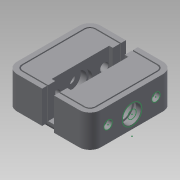
# Autodesk Inventor part: Sepatu
Saved by Autodesk Inventor 2015 SP1 (Build 190203100, 203)
## iProperties
Created: 2015-02-21
Part Number: Sepatu
Material: Generic
Document SubType Name: Modeling
Designer: Rafi Kurnia Putra
Density: 1 g/cm^3
Appearance: Default
Author: Rafi Kurnia Putra
Autodesk Inventor part; units mm, degrees
note: some values were not read from the file. Chosen so that the rebuilt part matches the saved one: copy form of "Mirror3".
ref_plane "YZ Plane" through (0, 0, 0) normal (1, 0, 0) x (0, 1, 0)
ref_plane "XZ Plane" through (0, 0, 0) normal (0, 1, 0) x (-1, 0, 0)
sketch "Sketch1" plane through (0, 0, 0) normal (0, 1, 0) x (-1, 0, 0)
  line L0 (-15, 15) -> (15, 15)
  line L1 (15, -15) -> (-15, -15)
  line L2 (-15, 15) -> (15, -15) construction
  line L3 (15, 15) -> (-15, -15) construction
  line L4 (15, 15) -> (15, 2.5)
  line L5 (15, -2.5) -> (15, -15)
  line L6 (-15, -15) -> (-15, -2.5)
  line L7 (-15, 2.5) -> (-15, 15)
  line L8 (12, 2.5) -> (12, 12)
  line L9 (12, 12) -> (-12, 12)
  line L10 (-12, 12) -> (-12, 2.5)
  line L11 (12, -2.5) -> (12, -12)
  line L12 (12, -12) -> (-12, -12)
  line L13 (-12, -12) -> (-12, -2.5)
  line L14 (15, 2.5) -> (12, 2.5)
  line L15 (15, -2.5) -> (12, -2.5)
  line L16 (-12, 2.5) -> (-15, 2.5)
  line L17 (-12, -2.5) -> (-15, -2.5)
  line L18 (12, 2.5) -> (12, -2.5)
  line L19 (-12, 2.5) -> (-12, -2.5)
  line L20 (15, -2.5) -> (15, 2.5)
  line L21 (-15, -2.5) -> (-15, 2.5)
  point P0 (0, 0)
  point P1 (15, -2.5)
  dimension "d0" = 30
  dimension "d1" = 30
  constraints: 44 end point, 9 parallel, 5 horizontal, 3 perpendicular, 2 midpoint, 2 vertical, 4 other
  measures "d0" distance of L1.start L1.end
  measures "d1" distance of L0.end L1.start
extrude "Extrusion1" add sketch "Sketch1" along normal blind 3 contours L10 L9 L8 L18 L11 L12 L13 L19
extrude "Extrusion2" add sketch "Sketch1" along normal blind 30 contours L0 L4 L14 L8 L9 L10 L16 L7 | L17 L13 L12 L11 L15 L5 L1 L6
extrude "Extrusion3" add sketch "Sketch1" along normal blind 3 contours L16 L19 L17 L21 | L20 L15 L18 L14
sketch "Sketch2" plane through (-15, 0, 15) normal (0, 0, 1) x (1, 0, 0)
  circle A0 centre (15, 8) radius 5
  line L0 (0, 0) -> (30, 0) projected
  circle A1 centre (15, 8) radius 1.75
  circle A2 centre (15, 8) radius 4.125
  dimension "d8" = 10
  dimension "d9" = 8
  dimension "d12" = 3.5
  dimension "d21" = 8.25
  constraints: 3 centre point, 2 coincident
  measures "d8" diameter of A0
  measures "d9" distance from line of L0 A0.centre
  measures "d12" diameter of A1
  measures "d21" diameter of A2
extrude "Extrusion6" add sketch "Sketch2" against normal blind 11 contours A0 | A1 | A2
extrude "Extrusion7" cut sketch "Sketch2" against normal up to next contours A1
extrude "Extrusion8" cut sketch "Sketch2" against normal blind 1.5 contours A0 | A2
extrude "Extrusion9" cut sketch "Sketch2" against normal blind 4 contours A1 | A2
fillet "Fillet1" radius 2 4 edges at (15, 0, 0) (0, 0, 15) (0, 0, -15) (-15, 0, 0)
fillet "Fillet2" radius 2 8 edges at (14.4142, 0.5858, 14.4142) (15, 16, 15) (14.4142, 0.5858, -14.4142) (15, 16, -15) (-14.4142, 0.5858, -14.4142) (-15, 16, -15) (-14.4142, 0.5858, 14.4142) (-15, 16, 15)
ref_plane "Work Plane1" through (0, 0, 9.5) normal (0, 0, 1) x (1, 0, 0)
mirror "Mirror3" about plane through (0, 0, 9.5) normal (0, 0, 1) of "Extrusion8", "Extrusion9", "Extrusion7" geometry pattern yes
mirror "Mirror4" about plane through (0, 0, 0) normal (0, 0, 1) of "Extrusion8", "Extrusion9", "Extrusion6", "Extrusion7", "Mirror3"
sketch "Sketch6" plane through (0, 30, 0) normal (0, 1, 0) x (1, 0, 0)
  line L0 (-15, -2.5) -> (-15, -13) projected
  arc A0 (-15, -13) -> (-13, -15) centre (-13, -13) ccw projected
  line L1 (-13, -15) -> (13, -15) projected
  arc A1 (13, -15) -> (15, -13) centre (13, -13) ccw projected
  line L2 (15, -13) -> (15, -2.5) projected
  line L3 (15, 2.5) -> (15, 13) projected
  arc A2 (15, 13) -> (13, 15) centre (13, 13) ccw projected
  line L4 (13, 15) -> (-13, 15) projected
  arc A3 (-13, 15) -> (-15, 13) centre (-13, 13) ccw projected
  line L5 (-15, 13) -> (-15, 2.5) projected
  line L6 (15.5, -2.5) -> (15.5, -13)
  arc A4 (13, -15.5) -> (15.5, -13) centre (13, -13) ccw
  line L7 (13, -15.5) -> (-13, -15.5)
  arc A5 (-15.5, -13) -> (-13, -15.5) centre (-13, -13) ccw
  line L8 (-15.5, -13) -> (-15.5, -2.5)
  line L9 (-15.5, 2.5) -> (-15.5, 13)
  arc A6 (-13, 15.5) -> (-15.5, 13) centre (-13, 13) ccw
  line L10 (-13, 15.5) -> (13, 15.5)
  arc A7 (15.5, 13) -> (13, 15.5) centre (13, 13) ccw
  line L11 (15.5, 13) -> (15.5, 2.5)
  line L12 (-17.5, -2.5) -> (-17.5, -13)
  arc A8 (-17.5, -13) -> (-13, -17.5) centre (-13, -13) ccw
  line L13 (-13, -17.5) -> (13, -17.5)
  arc A9 (13, -17.5) -> (17.5, -13) centre (13, -13) ccw
  line L14 (17.5, -13) -> (17.5, -2.5)
  line L15 (17.5, 2.5) -> (17.5, 13)
  arc A10 (17.5, 13) -> (13, 17.5) centre (13, 13) ccw
  line L16 (13, 17.5) -> (-13, 17.5)
  arc A11 (-13, 17.5) -> (-17.5, 13) centre (-13, 13) ccw
  line L17 (-17.5, 13) -> (-17.5, 2.5)
  line L18 (17.5, -2.5) -> (15.5, -2.5)
  line L19 (-15.5, -2.5) -> (-17.5, -2.5)
  line L20 (-15.5, 2.5) -> (-17.5, 2.5)
  line L21 (17.5, 2.5) -> (15.5, 2.5)
  point P0 (0, 0)
  dimension "d38" = 0.5
  dimension "d39" = 0.5
  dimension "d40" = 2
  dimension "d41" = 2
  constraints: 32 end point, 16 point on circle, 8 centre point, 2 horizontal, 1 parallel, 1 perpendicular, 16 other
  measures "d38" distance between parallel lines of L6 L2
  measures "d39" distance between parallel lines of L3 L11
  measures "d40" distance between parallel lines of L7 L13
  measures "d41" distance between parallel lines of L10 L16
extrude "Extrusion11" add sketch "Sketch6" against normal blind 27.5
sketch "Sketch10" plane through (-13, 30, 17.5) normal (0, 0, 1) x (1, 0, 0)
  line L0 (26, -27.5) -> (0, -27.5) projected
  circle A0 centre (13, -22) radius 1.75 projected
  line L1 (0, -30) -> (26, -30) projected
  line L2 (30.5, 0) -> (30.5, -27.5) projected
  line L3 (-4.5, 0) -> (30.5, 0)
  line L4 (30.5, 0) -> (30.5, -14)
  line L5 (30.5, -14) -> (-4.5, -14)
  line L6 (-4.5, -14) -> (-4.5, 0)
  point P0 (13, -30)
  point P1 (13, -14)
  dimension "d51" = 5.5
  dimension "d52" = 8
  constraints: 8 end point, 2 parallel, 1 horizontal, 1 perpendicular, 1 point on line
  measures "d51" distance from line of L0 A0.centre
  measures "d52" distance of point (13, -14) A0.centre
extrude "Extrusion15" cut sketch "Sketch10" against normal through all contours L2 L5 L6 L3
sketch "Sketch11" plane through (-13, 2.5, 17.5) normal (0, 0, 1) x (1, 0, 0)
  circle A0 centre (13, 5.5) radius 4.125 projected
  circle A1 centre (13, 5.5) radius 3.75
  point P0 (13, -2.5)
  dimension "d55" = 7.5
  constraints: 1 centre point, 1 coincident
  measures "d55" diameter of A1
extrude "Extrusion16" cut sketch "Sketch11" against normal blind 2 contours A1
mirror "Mirror7" about plane through (0, 0, 0) normal (0, 0, 1) of "Extrusion16"
sketch "Sketch12" plane through (13, 2.5, -17.5) normal (0, 0, -1) x (-1, 0, 0)
  circle A0 centre (13, 5.5) radius 3.75 projected
  line L0 (26, 13.5) -> (0, 13.5) projected
  line L1 (0, 13.5) -> (0, 0) projected
  line L2 (26, 0) -> (0, 0) projected
  line L3 (26, 13.5) -> (26, 0) projected
  line L4 (0, 13.5) -> (26, 0) construction
  line L5 (26, 0) -> (26, 13.5)
  line L6 (26, 13.5) -> (26, 0) projected
  line L7 (26, 13.5) -> (0, 0) construction
  line L8 (0, 0) -> (13, 6.75) construction
  line L9 (13, 12.25) -> (13, 6.75) construction
  line L10 (-2, 0.5) -> (1, 0.5) projected
  line L11 (13, 6.75) -> (19, 6.75) construction
  circle A1 centre (3, 6.75) radius 1.75
  circle A2 centre (23, 6.75) radius 1.75
  point P0 (13, -2.5)
  dimension "d61" = 3.5
  constraints: 12 end point, 2 centre point, 2 perpendicular, 1 collinear, 1 midpoint, 1 symmetric about line, 1 other
  measures "d61" diameter of A1
extrude "Extrusion17" cut sketch "Sketch12" against normal through all contours A1 | A2
sketch "Sketch13" plane through (-12, 3, -12) normal (0, 0, 1) x (1, 0, 0)
  circle A0 centre (22, 6.25) radius 1.75 projected
  circle A1 centre (2, 6.25) radius 1.75 projected
  line L0 (24, 13) -> (0, 13) projected
  line L1 (0, 0) -> (0, 13) projected
  line L2 (12, 0) -> (0, 0) projected
  circle A2 centre (12, 5) radius 5 projected
  line L3 (24, 0) -> (12, 0) projected
  line L4 (24, 0) -> (24, 13) projected
  point P0 (12, -3)
  constraints: 1 vertical alignment
extrude "Extrusion18" add sketch "Sketch13" along normal blind 8
mirror "Mirror8" about plane through (0, 0, 0) normal (0, 0, 1) of "Extrusion18"
sketch "Sketch14" plane through (-13, 2.5, 17.5) normal (0, 0, 1) x (1, 0, 0)
  circle A0 centre (3, 6.75) radius 1.75 projected
  circle A1 centre (13, 5.5) radius 1.75 projected
  circle A2 centre (13, 5.5) radius 4.125 projected
  circle A3 centre (23, 6.75) radius 1.75 projected
  point P0 (13, -2.5)
body "Solid1"
